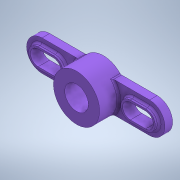
# Autodesk Inventor part: P01_Marcos_Uriel_Martinez_Ortiz
Saved by Autodesk Inventor 2021 (Build 250183000, 183)
## iProperties
Created: 2021-03-12
Part Number: P01_Marcos_Uriel_Martinez_Ortiz
Material: Steel ASTM A36
Document SubType Name: Modeling
Designer: uriel
Mass: 853.796 g
Surface Area: 268.517 cm^2
Volume: 108.764 cm^3
Density: 7.85 g/cm^3
Appearance: Violet
Author: uriel
Autodesk Inventor part; units mm, degrees
ref_plane "YZ Plane" through (0, 0, 0) normal (1, 0, 0) x (0, 1, 0)
ref_plane "XZ Plane" through (0, 0, 0) normal (0, 1, 0) x (-1, 0, 0)
ref_plane "XY Plane" through (0, 0, 0) normal (0, 0, 1) x (1, 0, 0)
sketch "Sketch1" plane through (0, 0, 0) normal (0, 0, 1) x (1, 0, 0)
  line L0 (-18.363138, 0) -> (121.636862, 0) construction
  arc A0 (-18.363138, 20) -> (-18.363138, -20) centre (-18.363138, 0) ccw
  arc A1 (121.636862, -20) -> (121.636862, 20) centre (121.636862, 0) ccw
  line L1 (121.636862, 0) -> (101.636862, 0) construction
  line L2 (121.636862, 10) -> (101.636862, 10)
  line L3 (101.636862, -10) -> (121.636862, -10)
  arc A2 (121.636862, -10) -> (121.636862, 10) centre (121.636862, 0) ccw
  arc A3 (101.636862, 10) -> (101.636862, -10) centre (101.636862, 0) ccw
  line L4 (-18.363138, 0) -> (1.636862, 0) construction
  line L5 (-18.363138, -10) -> (1.636862, -10)
  line L6 (1.636862, 10) -> (-18.363138, 10)
  arc A4 (-18.363138, 10) -> (-18.363138, -10) centre (-18.363138, 0) ccw
  arc A5 (1.636862, -10) -> (1.636862, 10) centre (1.636862, 0) ccw
  circle A6 centre (51.636862, 0) radius 15
  line L7 (121.636862, 20) -> (73.997541, 20)
  line L8 (29.276182, 20) -> (-18.363138, 20)
  line L9 (-18.363138, -20) -> (29.276182, -20)
  line L10 (73.997541, -20) -> (121.636862, -20)
  arc A7 (73.997541, 20) -> (29.276182, 20) centre (51.636862, 0) ccw
  arc A8 (29.276182, -20) -> (73.997541, -20) centre (51.636862, 0) ccw
  point P0 (0, 0)
  point P1 (111.636862, 0)
  point P2 (-8.363138, 0)
  dimension "d0" = 40
  dimension "d1" = 140
  dimension "d2" = 20
  dimension "d3" = 20
  dimension "d4" = 20
  dimension "d5" = 20
  dimension "d7" = 30
  constraints: 28 end point, 16 point on circle, 16 tangent, 9 centre point, 6 parallel, 3 midpoint, 2 coincident, 2 point on line, 1 horizontal
  measures "d0" diameter of A1
  measures "d1" distance of L7.start L8.end
  measures "d2" diameter of A3
  measures "d3" distance of L2.start L2.end
  measures "d4" distance of L0.start L4.end
  measures "d5" diameter of A5
  measures "d7" diameter of A6
sketch "Sketch1 outline for Extrusion1" plane through (0, 0, 0) normal (0, 0, 1) x (1, 0, 0)
  arc A0 (-18.363138, 20) -> (-18.363138, -20) centre (-18.363138, 0) ccw
  line L0 (29.276182, 20) -> (-18.363138, 20)
  line L1 (-18.363138, -20) -> (29.276182, -20)
  arc A1 (73.997541, 20) -> (29.276182, 20) centre (51.636862, 0) ccw
  arc A2 (29.276182, -20) -> (73.997541, -20) centre (51.636862, 0) ccw
  line L2 (121.636862, 20) -> (73.997541, 20)
  line L3 (73.997541, -20) -> (121.636862, -20)
  arc A3 (121.636862, -20) -> (121.636862, 20) centre (121.636862, 0) ccw
  arc A4 (-18.363138, -10) -> (-18.363138, 10) centre (-18.363138, 0) cw
  line L4 (1.636862, -10) -> (-18.363138, -10)
  arc A5 (1.636862, 10) -> (1.636862, -10) centre (1.636862, 0) cw
  line L5 (-18.363138, 10) -> (1.636862, 10)
  circle A6 centre (51.636862, 0) radius 15
  arc A7 (121.636862, 10) -> (121.636862, -10) centre (121.636862, 0) cw
  line L6 (101.636862, 10) -> (121.636862, 10)
  arc A8 (101.636862, -10) -> (101.636862, 10) centre (101.636862, 0) cw
  line L7 (121.636862, -10) -> (101.636862, -10)
extrude "Extrusion1" add sketch "Sketch1 outline for Extrusion1" along normal blind 10
sketch "Sketch2" plane through (0, 0, 10) normal (0, 0, 1) x (1, 0, 0)
  line L0 (-18.363138, 10) -> (1.636862, 10)
  arc A0 (1.636862, -10) -> (1.636862, 10) centre (1.636862, 0) ccw
  line L1 (1.636862, -10) -> (-18.363138, -10)
  arc A1 (-18.363138, 10) -> (-18.363138, -10) centre (-18.363138, 0) ccw
  arc A2 (101.636862, 10) -> (101.636862, -10) centre (101.636862, 0) ccw
  line L2 (101.636862, 10) -> (121.636862, 10)
  arc A3 (121.636862, -10) -> (121.636862, 10) centre (121.636862, 0) ccw
  line L3 (121.636862, -10) -> (101.636862, -10)
  line L4 (1.636862, 12.5) -> (-18.363138, 12.5)
  arc A4 (-18.363138, 12.5) -> (-18.363138, -12.5) centre (-18.363138, 0) ccw
  line L5 (-18.363138, -12.5) -> (1.636862, -12.5)
  arc A5 (1.636862, -12.5) -> (1.636862, 12.5) centre (1.636862, 0) ccw
  line L6 (121.636862, 12.5) -> (101.636862, 12.5)
  arc A6 (101.636862, 12.5) -> (101.636862, -12.5) centre (101.636862, 0) ccw
  line L7 (101.636862, -12.5) -> (121.636862, -12.5)
  arc A7 (121.636862, -12.5) -> (121.636862, 12.5) centre (121.636862, 0) ccw
  point P0 (0, 0)
  dimension "d10" = 2.5
  dimension "d11" = 2.5
  constraints: 8 end point, 8 point on circle, 4 centre point, 6 other
  measures "d10" radial gap between concentric circles of A0 A5
  measures "d11" distance between parallel lines of L2 L6
sketch "Sketch2 outline for Extrusion2" plane through (0, 0, 10) normal (0, 0, 1) x (1, 0, 0)
  line L0 (121.636862, 12.5) -> (101.636862, 12.5)
  arc A0 (121.636862, -12.5) -> (121.636862, 12.5) centre (121.636862, 0) ccw
  arc A1 (101.636862, 12.5) -> (101.636862, -12.5) centre (101.636862, 0) ccw
  line L1 (101.636862, -12.5) -> (121.636862, -12.5)
  line L2 (121.636862, -10) -> (101.636862, -10)
  arc A2 (121.636862, 10) -> (121.636862, -10) centre (121.636862, 0) cw
  line L3 (101.636862, 10) -> (121.636862, 10)
  arc A3 (101.636862, -10) -> (101.636862, 10) centre (101.636862, 0) cw
  line L4 (1.636862, 12.5) -> (-18.363138, 12.5)
  arc A4 (1.636862, -12.5) -> (1.636862, 12.5) centre (1.636862, 0) ccw
  arc A5 (-18.363138, 12.5) -> (-18.363138, -12.5) centre (-18.363138, 0) ccw
  line L5 (-18.363138, -12.5) -> (1.636862, -12.5)
  line L6 (1.636862, -10) -> (-18.363138, -10)
  arc A6 (1.636862, 10) -> (1.636862, -10) centre (1.636862, 0) cw
  line L7 (-18.363138, 10) -> (1.636862, 10)
  arc A7 (-18.363138, -10) -> (-18.363138, 10) centre (-18.363138, 0) cw
extrude "Extrusion2" add sketch "Sketch2 outline for Extrusion2" along normal blind 5
sketch "Sketch3" plane through (0, 0, 10) normal (0, 0, 1) x (1, 0, 0)
  circle A0 centre (51.636862, 0) radius 15
  arc A1 (29.276182, -20) -> (73.997541, -20) centre (51.636862, 0) ccw
  circle A2 centre (51.636862, 0) radius 30
  circle A3 centre (51.636862, 0) radius 15.36853
  point P0 (0, 0)
  point P1 (29.276182, -20)
  constraints: 2 coincident, 1 centre point, 3 other
sketch "Sketch3 outline for Extrusion3" plane through (0, 0, 10) normal (0, 0, 1) x (1, 0, 0)
  arc A0 (73.997541, -20) -> (29.276182, -20) centre (51.636862, 0) ccw
  arc A1 (29.276182, -20) -> (73.997541, -20) centre (51.636862, 0) ccw
  circle A2 centre (51.636862, 0) radius 15.36853
extrude "Extrusion3" add sketch "Sketch3 outline for Extrusion3" along normal blind 25
fillet "Fillet1" radius 2.5 14 edges at (21.6369, 0, 10) (29.2762, -20, 5) (-30.8631, 0, 10) (-8.3631, 12.5, 10) (14.1369, 0, 10) (-8.3631, -12.5, 10) (89.1369, 0, 10) (111.6369, 12.5, 10) (134.1369, 0, 10) (111.6369, -12.5, 10) (81.6369, 0, 10) (73.9975, -20, 5) (73.9975, 20, 5) (29.2762, 20, 5)
body "Solid1"
